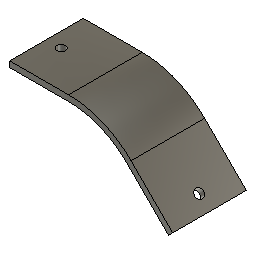
Test_Object_Fusion (Autodesk Fusion 360 design; units mm, degrees)
Autodesk Fusion 360 part; units mm, degrees
sketch "Cross-section" plane through (0, 0, 0) normal (0, 1, 0) x (1, 0, 0)
  line L0 (0, 0) -> (0, -30) construction
  line L1 (0, 0) -> (21.2132, -21.2132) construction
  arc A0 (0, -30) -> (21.2132, -21.2132) centre (0, 0) ccw
  line L2 (0, -30) -> (-20, -30)
  line L3 (21.2132, -21.2132) -> (35.3553, -7.0711)
  line L4 (19.799, -19.799) -> (33.9411, -5.6569)
  arc A1 (0, -28) -> (19.799, -19.799) centre (0, 0) ccw
  line L5 (0, -28) -> (-20, -28)
  line L6 (-20, -28) -> (-20, -30)
  line L7 (33.9411, -5.6569) -> (35.3553, -7.0711)
  line L8 (0, -29) -> (-15, -29)
  line L9 (21.2132, -21.2132) -> (31.8198, -10.6066)
  dimension "d1" = 60
  dimension "d2" = 45
  dimension "d3" = 20
  dimension "d4" = 20
  dimension "d5" = -2
  dimension "d8" = 15
  dimension "d9" = 15
  constraint coincident L0.start L1.start
  constraint vertical L0
  constraint tangent A0 L2
  constraint tangent A0 L3
  constraint perpendicular L2 L6
  constraint perpendicular L4 L7
  constraint coincident L0 L8.start
  constraint perpendicular L0 L8
  constraint tangent A0 L9
  measures "d1" diameter of A0
  measures "d2" angle of L0 L1
  measures "d3" distance of L0.end L2.end
  measures "d4" distance of L1.end L3.end
  measures "d8" distance of L8.start L8.end
  measures "d9" distance of L1.end L9.end
extrude "Extrude1" add sketch "Cross-section" along normal blind 25
sketch "Mounting_hole_1" plane through (0, 0, 30) normal (0, 0, 1) x (-1, 0, 0)
  line L0 (20, 0) -> (0, 0)
  line L1 (0, 0) -> (0, -25)
  line L2 (0, -25) -> (20, -25)
  line L3 (20, -25) -> (20, 0)
  line L4 (0, -12.5) -> (15, -12.5)
  circle A0 centre (15, -12.5) radius 1.5
  dimension "d10" = 15
  dimension "d11" = 3
  constraint midpoint L1 L4.start
  constraint perpendicular L1 L4
  constraint coincident L4.end A0.centre
  measures "d10" distance of L4.start L4.end
  measures "d11" diameter of A0
extrude "Extrude2" cut sketch "Mounting_hole_1" against normal blind 6 contours A0
sketch "Mounting_hole_2" plane through (21.2132, 0, 21.2132) normal (0.707107, 0, 0.707107) x (0, 1, 0)
  line L0 (0, 0) -> (0, -20)
  line L1 (0, -20) -> (25, -20)
  line L2 (25, -20) -> (25, 0)
  line L3 (25, 0) -> (0, 0)
  line L4 (12.5, 0) -> (12.5, -15)
  circle A0 centre (12.5, -15) radius 1.5
  dimension "d14" = 15
  dimension "d15" = 3
  constraint midpoint L3 L4.start
  constraint perpendicular L3 L4
  constraint coincident L4.end A0.centre
  measures "d14" distance of L4.start L4.end
  measures "d15" diameter of A0
extrude "Extrude3" cut sketch "Mounting_hole_2" against normal blind 8 contours A0
named bodies: "Test_Object"
